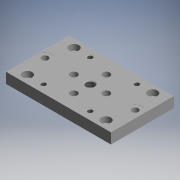
# Autodesk Inventor part: 1558863 EAGF-V2-KF-100---(J)
Saved by Autodesk Inventor 2017.3 (Build 213256000, 256)
## iProperties
Part Number: 1558863 EAGF-V2-KF-100---(J)
Material: Generic
Catalog Web Link: www.cadenas.de
Description: EAGF-V2-KF-(J)-Jochplatte
Vendor: FESTO
Document SubType Name: Modeling
Designer: partserver
Manufacturer: FESTO
Mass: 428.55 g
Surface Area: 706.736 cm^2
Volume: 428.55 cm^3
Density: 1 g/cm^3
Appearance: PSOLRGB-192-192-192
Category: PARTsolutions
Company: FESTO
Title: 1558863 EAGF-V2-KF-100---(J)
Author: Cadenas PARTsolutions
Comments: Jochplatte
PSOL_IDENT_0: {$CADENAS_DATA\23d-libs\festo\parts\e\eagf\parts\eagf_joch.prj},204 {VTYP=3D},{NB=1558863 EAGF-V2-KF
PSOL_IDENT_1: -100---(J)},{LINA=1558863 EAGF-V2-KF-100---(J)},{NN=EAGF-V2-KF-(J)},{DATE=20.07.2020 13:53:58},{GEOM
PSOL_IDENT_2: DATE=17.05.2016 09:08:00},{VERSION=},{LINEID=30},{WBVAR=},{WBNUMERIC=}  {NB=1558863 EAGF-V2-KF-100--
PSOL_IDENT_3: -(J)},{LINA=1558863 EAGF-V2-KF-100---(J)},{KT=DUMMY},{TNR=1558863},{TYP=EAGF-V2-KF-100},{KDM=100},{B=
PSOL_IDENT_4: 20.000},{D1=18.000},{D2=62.000},{D3=20.000},{D4=12.300},{D5=20.000},{D6=13.500},{D7=10.000},{D7P=1.5
PSOL_IDENT_5: 00},{D8=18.000},{D9=11.000},{D10=26.000},{D11=0.000},{H1=120.000},{H2=89.000},{L1=200.000},{L2=172.0
PSOL_IDENT_6: 00},{L3=150.000},{L4=89.000},{L5=0.000},{T1=8.500},{T2=13.000},{T3=11.000},{ANZ=4.000},{W=90.000}
NB: 1558863 EAGF-V2-KF-100---(J)
NN: EAGF-V2-KF-(J)
NT: Jochplatte
NBSYN: $TNR. $TYP.---(J)
LINA: 1558863 EAGF-V2-KF-100---(J)
CATALOG: Festo
TNR: 1558863
TYP: EAGF-V2-KF-100
KDM: 100
B: 20
D1: 18
D2: 62
D3: 20
D4: 12.3
D5: 20
D6: 13.5
D7: 10
D7P: 1.5
D8: 18
D9: 11
D10: 26
D11: 0
H1: 120
H2: 89
L1: 200
L2: 172
L3: 150
L4: 89
L5: 0
T1: 8.5
T2: 13
T3: 11
ANZ: 4
W: 90
SUPPLIER: FESTO
ARTICLENO: 1558863 EAGF-V2-KF-100---(J)
BOMINFO: 1558863 EAGF-V2-KF-100---(J)
CREATOR: CADENAS GmbH
Autodesk Inventor part; units mm, degrees
sketch "Sketch_1" plane through (0, 0, 0) normal (0, 0, 1) x (1, 0, 0)
  line L0 (-100, 60) -> (-100, -60)
  line L1 (-100, -60) -> (100, -60)
  line L2 (100, -60) -> (100, 60)
  line L3 (100, 60) -> (-100, 60)
  constraints: 8 end point
extrude "Extrusion1" add sketch "Sketch_1" against normal blind 20
sketch "Sketch_2" plane through (0, 0, 0) normal (1, 0, 0) x (0, 1, 0)
  line L0 (0, -20) -> (0, 0)
  line L1 (0, 0) -> (9, 0)
  line L2 (9, 0) -> (7.647, -1.353)
  line L3 (7.647, -1.353) -> (7.647, -18.647)
  line L4 (7.647, -18.647) -> (9, -20)
  line L5 (9, -20) -> (0, -20)
  line L6 (0, -20) -> (0, 0)
  constraints: 14 end point
revolve "Revolution1" cut sketch "Sketch_2" angle 360 about axis through (0, 0, -20) along (0, 0, -1)
thread "Thread1" size "M18x2.5" class "6H" standard "ISO Metric profile" full length
sketch "Sketch3" plane through (0, 0, 0) normal (0, 0, 1) x (1, 0, 0)
  point P0 (0, 31)
hole "Hole1" at (0, 31, 0) direction (0, 0, -1) diameter 13.5 depth 20 counterbore diameter 20 counterbore depth 13
pattern_linear "Rectangular Pattern1" count 2 spacing 43.8406 along (-0.7071068, -0.7071068, 0) count 2 spacing 43.8406 along (0.7071068, -0.7071068, 0) of "Hole1"
sketch "Sketch_5" plane through (44.5, 0, 0) normal (1, 0, 0) x (0, 0, -1)
  line L0 (20, 44.5) -> (0, 44.5)
  line L1 (0, 44.5) -> (0, 49.5)
  line L2 (0, 49.5) -> (0.812, 48.688)
  line L3 (0.812, 48.688) -> (19.188, 48.688)
  line L4 (19.188, 48.688) -> (20, 49.5)
  line L5 (20, 49.5) -> (20, 44.5)
  line L6 (20, 44.5) -> (0, 44.5)
  constraints: 14 end point
revolve "Revolution2" cut sketch "Sketch_5" angle 360 about axis through (44.5, 44.5, -20) along (0, 0, -1)
thread "Thread2" size "M10x1.5" class "6H" standard "ISO Metric profile" full length
pattern_linear "Rectangular Pattern2" count 2 spacing 89 along (-1, 0, 0) count 2 spacing 89 along (0, -1, 0) of "Revolution2"
sketch "Sketch5" plane through (0, 0, -20) normal (0, 0, -1) x (-1, 0, 0)
  point P0 (-75, 44.5)
  dimension "d14" = 43.8406
hole "Hole2" at (75, 44.5, -20) direction (0, 0, 1) diameter 11 depth 20 counterbore diameter 18 counterbore depth 11
pattern_linear "Rectangular Pattern3" count 2 spacing 150 along (-1, 0, 0) count 2 spacing 89 along (0, -1, 0) of "Hole2"
sketch "Sketch_9" plane through (0, 0, 0) normal (0, 1, 0) x (-1, 0, 0)
  line L0 (-86, 0) -> (-86, -20)
  line L1 (-86, -20) -> (-99, -20)
  line L2 (-99, -20) -> (-99, -19.8)
  line L3 (-99, -19.8) -> (-92.15, -19.8)
  line L4 (-92.15, -19.8) -> (-92.15, -8.5)
  line L5 (-92.15, -8.5) -> (-96, -8.5)
  line L6 (-96, -8.5) -> (-96, 0)
  line L7 (-96, 0) -> (-86, 0)
  line L8 (-86, 0) -> (-86, -20)
  constraints: 18 end point
revolve "Revolution3" cut sketch "Sketch_9" angle 360 about axis through (86, 0, 0) along (0, 0, 1)
sketch "Sketch_10" plane through (0, 0, 0) normal (0, 1, 0) x (-1, 0, 0)
  line L0 (86, 0) -> (86, -20)
  line L1 (86, -20) -> (73, -20)
  line L2 (73, -20) -> (73, -19.8)
  line L3 (73, -19.8) -> (79.85, -19.8)
  line L4 (79.85, -19.8) -> (79.85, -8.5)
  line L5 (79.85, -8.5) -> (76, -8.5)
  line L6 (76, -8.5) -> (76, 0)
  line L7 (76, 0) -> (86, 0)
  line L8 (86, 0) -> (86, -20)
  constraints: 18 end point
revolve "Revolution4" cut sketch "Sketch_10" angle 360 about axis through (-86, 0, 0) along (0, 0, 1)
ref_plane "ANBAU_XY" through (0, 0, 0) normal (0, 0, 1) x (1, 0, 0)
ref_plane "ANBAU_YZ" through (0, 0, 0) normal (1, 0, 0) x (0, 1, 0)
ref_plane "ANBAU_ZX" through (0, 0, 0) normal (0, 1, 0) x (0, 0, 1)
ref_plane "DIN6912_1_XY" through (86, 0, -8.5) normal (0, 0, -1) x (1, 0, 0)
ref_plane "DIN6912_1_YZ" through (86, 0, -8.5) normal (1, 0, 0) x (0, -1, 0)
ref_plane "DIN6912_1_ZX" through (86, 0, -8.5) normal (0, -1, 0) x (0, 0, -1)
ref_plane "DIN6912_2_XY" through (-86, 0, -8.5) normal (0, 0, -1) x (1, 0, 0)
ref_plane "DIN6912_2_YZ" through (-86, 0, -8.5) normal (1, 0, 0) x (0, -1, 0)
ref_plane "DIN6912_2_ZX" through (-86, 0, -8.5) normal (0, -1, 0) x (0, 0, -1)
ref_plane "DIN913_IP1_XY" through (0, 0, 0) normal (0, 0, 1) x (1, 0, 0)
ref_plane "DIN913_IP1_YZ" through (0, 0, 0) normal (1, 0, 0) x (0, 1, 0)
ref_plane "DIN913_IP1_ZX" through (0, 0, 0) normal (0, 1, 0) x (0, 0, 1)
ref_plane "GS_XY" through (0, 0, -20) normal (0, 0, 1) x (1, 0, 0)
ref_plane "GS_YZ" through (0, 0, -20) normal (1, 0, 0) x (0, 1, 0)
ref_plane "GS_ZX" through (0, 0, -20) normal (0, 1, 0) x (0, 0, 1)
ref_plane "RING_XY" through (0, 0, -20) normal (0, 0, -1) x (1, 0, 0)
ref_plane "RING_YZ" through (0, 0, -20) normal (1, 0, 0) x (0, -1, 0)
ref_plane "RING_ZX" through (0, 0, -20) normal (0, -1, 0) x (0, 0, -1)
ref_plane "SCREW_1_XY" through (0, 31, -13) normal (0, 0, 1) x (1, 0, 0)
ref_plane "SCREW_1_YZ" through (0, 31, -13) normal (1, 0, 0) x (0, 1, 0)
ref_plane "SCREW_1_ZX" through (0, 31, -13) normal (0, 1, 0) x (0, 0, 1)
ref_plane "SCREW_2_XY" through (-31, 0, -13) normal (0, 0, 1) x (1, 0, 0)
ref_plane "SCREW_2_YZ" through (-31, 0, -13) normal (1, 0, 0) x (0, 1, 0)
ref_plane "SCREW_2_ZX" through (-31, 0, -13) normal (0, 1, 0) x (0, 0, 1)
ref_plane "SCREW_3_XY" through (0, -31, -13) normal (0, 0, 1) x (1, 0, 0)
ref_plane "SCREW_3_YZ" through (0, -31, -13) normal (1, 0, 0) x (0, 1, 0)
ref_plane "SCREW_3_ZX" through (0, -31, -13) normal (0, 1, 0) x (0, 0, 1)
ref_plane "SCREW_4_XY" through (31, 0, -13) normal (0, 0, 1) x (1, 0, 0)
ref_plane "SCREW_4_YZ" through (31, 0, -13) normal (1, 0, 0) x (0, 1, 0)
ref_plane "SCREW_4_ZX" through (31, 0, -13) normal (0, 1, 0) x (0, 0, 1)
ref_plane "STANGE_XY" through (86, 0, -19.8) normal (0, 0, 1) x (1, 0, 0)
ref_plane "STANGE_YZ" through (86, 0, -19.8) normal (1, 0, 0) x (0, 1, 0)
ref_plane "STANGE_ZX" through (86, 0, -19.8) normal (0, 1, 0) x (0, 0, 1)
ref_plane "STANGE_2_XY" through (-86, 0, -19.8) normal (0, 0, 1) x (1, 0, 0)
ref_plane "STANGE_2_YZ" through (-86, 0, -19.8) normal (1, 0, 0) x (0, 1, 0)
ref_plane "STANGE_2_ZX" through (-86, 0, -19.8) normal (0, 1, 0) x (0, 0, 1)
body "Solid1"
